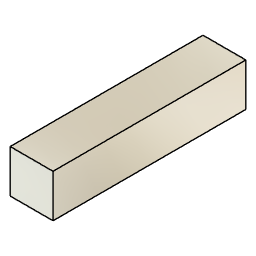
Loadcell1 (Autodesk Fusion 360 design; units mm, degrees)
Autodesk Fusion 360 part; units mm, degrees
sketch "Sketch1" plane through (0, 0, 0) normal (1, 0, 0) x (0, 1, 0) in component "Component"
  line L0 (0, 0) -> (54, 0)
  line L1 (54, 0) -> (54, 12)
  line L2 (54, 12) -> (0, 12)
  line L3 (0, 12) -> (0, 0)
  dimension "d1_2" = 12
  dimension "d2_2" = 54
  constraint horizontal L0
  constraint vertical L1
  constraint horizontal L2
  constraint vertical L3
  constraint coincident L0.start L3.end
  measures "d1_2" distance of L0.start L2.end
  measures "d2_2" distance of L1.end L2.end
extrude "Extrude1" add sketch "Sketch1" along normal blind 12 in component "Component"
component "Component" placed x (1, 0, 0) y (0, 1, 0) z (0, 0, 1) at (0, 0, 0)
